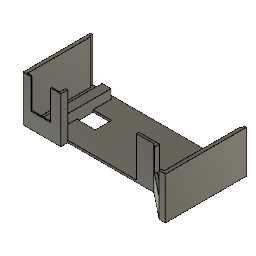
Box_gap_part1 v2 (Autodesk Fusion 360 design; units mm, degrees)
Autodesk Fusion 360 part; units mm, degrees
note: some values were not read from the file. Set by a fixed rule: which sketch regions a step uses.
sketch "草图1" plane through (0, 0, 0) normal (0, 1, 0) x (1, 0, 0)
  line L0 (0, 0) -> (56, 0)
  line L1 (56, 0) -> (56, -136)
  line L2 (56, -136) -> (0, -136)
  line L3 (0, -136) -> (0, 0)
  line L4 (3, -3) -> (53, -3)
  line L5 (53, -3) -> (53, -133)
  line L6 (53, -133) -> (3, -133)
  line L7 (3, -133) -> (3, -3)
  dimension "d1" = 136
  dimension "d2" = 56
  dimension "d3" = 3
  dimension "d4" = 3
  dimension "d5" = 3
  dimension "d6" = 3
  constraint horizontal L0
  constraint vertical L1
  constraint horizontal L2
  constraint vertical L3
  constraint coincident L0.start L3.end
  constraint horizontal L4
  constraint vertical L5
  constraint horizontal L6
  constraint vertical L7
  measures "d1" distance of L0.end L1.end
  measures "d2" distance of L1.end L2.end
  measures "d3" distance of L2 L6
  measures "d4" distance of L0 L4
  measures "d5" distance of L1 L5
  measures "d6" distance of L3 L7
extrude "拉伸1" add sketch "草图1" along normal blind 53
sketch "草图2" plane through (56, 0, 0) normal (1, 0, 0) x (0, 1, 0)
  line L0 (0, 136) -> (0, 0)
  line L1 (0, 0) -> (53, 0)
  line L2 (53, 0) -> (53, 136)
  line L3 (53, 136) -> (0, 136)
  line L4 (0, 0) -> (0, 28)
  line L5 (-16, 5) -> (0, 25)
  line L6 (0, 0) -> (-18, 0)
  line L7 (-18, 0) -> (-18, 5.5)
  line L8 (-18, 5.5) -> (0, 28)
  line L9 (0, 3) -> (-16, 3)
  line L10 (-16, 3) -> (-16, 5)
  point P0 (0, 3)
  dimension "d9" = 28
  dimension "d13" = 16
  dimension "d14" = 18
  constraint coincident L0.end L1.start
  constraint coincident L0 L4.end
  constraint perpendicular L1 L4
  constraint coincident L4 L5.end
  constraint perpendicular L4 L6
  constraint coincident P0 L9.start
  constraint perpendicular L4 L9
  measures "d9" distance of L0.end L4.end
  measures "d13" distance of P0 L9.end
  measures "d14" distance of L0.end L6.end
extrude "拉伸2" add sketch "草图2" against normal blind 56 contours L0 L4 L5 L6 L7 L8 L9 L10
sketch "草图3" plane through (0, 0, 0) normal (1, 0, 0) x (0, 1, 0)
  line L0 (0, 0) -> (0, 28)
  line L1 (0, 25) -> (0, 3)
  line L2 (-16, 3) -> (0, 3)
  line L3 (-16, 3) -> (-16, 5)
  line L4 (-16, 5) -> (0, 25)
  point P0 (0, 25)
  point P1 (0, 3)
  point P2 (-16, 3)
  point P3 (-16, 5)
  point P4 (0, 25)
  constraint coincident P4 P0
  constraint coincident P1 L1.end
  constraint coincident P2 L2.start
  constraint coincident P3 L3.end
extrude "拉伸3" add sketch "草图3" along normal blind 3
sketch "草图4" plane through (56, 0, 0) normal (1, 0, 0) x (0, 1, 0)
  line L0 (0, 25) -> (0, 3)
  line L1 (0, 3) -> (-16, 3)
  line L2 (-16, 3) -> (-16, 5)
  line L3 (-16, 5) -> (0, 25)
  line L4 (0, 28) -> (-18, 5.5)
  line L5 (-18, 5.5) -> (-18, 0)
  line L6 (-18, 0) -> (53, 0)
  line L7 (53, 0) -> (53, 136)
  line L8 (53, 136) -> (0, 136)
  line L9 (0, 136) -> (0, 28)
  line L10 (0, 25) -> (0, 3)
  line L11 (-16, 5) -> (0, 25)
  constraint coincident L0.start L3.end
  constraint coincident L0.end L1.start
  constraint coincident L2.end L3.start
extrude "拉伸4" add sketch "草图4" against normal blind 3 contours L0 L1 L2 L3 L10 L11
sketch "草图5" plane through (0, 0, 0) normal (0, -1, 0) x (1, 0, 0)
  line L0 (53, 28) -> (56, 28)
  line L1 (56, 28) -> (56, 136)
  line L2 (56, 136) -> (0, 136)
  line L3 (0, 136) -> (0, 28)
  line L4 (0, 28) -> (3, 28)
  line L5 (3, 28) -> (3, 133)
  line L6 (3, 133) -> (53, 133)
  line L7 (53, 133) -> (53, 28)
  line L8 (53, 25) -> (3, 25)
  line L9 (3, 25) -> (3, 45)
  line L10 (3, 45) -> (53, 45)
  line L11 (53, 45) -> (53, 25)
  point P0 (53, 25)
  dimension "d21" = 20
  constraint horizontal L8
  constraint vertical L9
  constraint horizontal L10
  constraint vertical L11
  constraint coincident L5 L9.end
  constraint coincident P0 L8.start
  measures "d21" distance of P0 L10.end
extrude "拉伸7" add sketch "草图5" against normal blind 2 contours L5 L7 L8 L9 L10 L11
extrude "拉伸5" add sketch "草图5" against normal blind 2 contours L5 L7 L8 L9 L10 L11
sketch "草图7" plane through (0, -18, 0) normal (0, -1, 0) x (1, 0, 0)
  line L0 (56, 0) -> (56, 5.5)
  line L1 (56, 5.5) -> (0, 5.5)
  line L2 (0, 5.5) -> (0, 0)
  line L3 (0, 0) -> (56, 0)
  line L4 (18, 3) -> (38, 3)
  line L5 (38, 3) -> (38, 25)
  line L6 (38, 25) -> (18, 25)
  line L7 (18, 25) -> (18, 3)
  line L8 (3, 3) -> (53, 3)
  line L9 (53, 25) -> (3, 25)
  dimension "d26" = 15
  dimension "d27" = 15
  constraint horizontal L4
  constraint vertical L5
  constraint horizontal L6
  constraint vertical L7
  constraint coincident L5.end L9
  constraint coincident L4.start L8
  measures "d26" distance of L4.start L8.start
  measures "d27" distance of L4.end L8.end
extrude "拉伸6" cut sketch "草图7" against normal blind 20 contours L1 L5 L6 L7 L9
sketch "草图8" plane through (56, 0, 0) normal (1, 0, 0) x (0, 1, 0)
  line L0 (0, 28) -> (-18, 5.5)
  line L1 (-18, 5.5) -> (-18, 0)
  line L2 (-18, 0) -> (53, 0)
  line L3 (53, 0) -> (53, 136)
  line L4 (53, 136) -> (0, 136)
  line L5 (0, 136) -> (0, 28)
  line L6 (0, 136) -> (-6, 136)
  line L7 (0, 133) -> (-5, 133)
  line L8 (-5, 133) -> (-5, 105)
  line L9 (-5, 105) -> (0, 105)
  line L10 (-6, 136) -> (-6, 103)
  line L11 (-6, 103) -> (0, 102.9799)
  point P0 (0, 136)
  point P1 (0, 133)
  dimension "d32" = 6
  dimension "d36" = 28
  dimension "d37" = 5
  dimension "d38" = 33
  constraint coincident P0 L4.end
  constraint perpendicular L5 L6
  constraint coincident P1 L7.start
  constraint perpendicular L5 L7
  constraint perpendicular L7 L8
  constraint coincident L5 L9.end
  constraint perpendicular L8 L9
  constraint perpendicular L6 L10
  constraint coincident L5 L11.end
  measures "d32" distance of L6.end P0
  measures "d36" distance of L7.end L8.end
  measures "d37" distance of L8 L9.end
  measures "d38" distance of L6.end L10.end
extrude "拉伸8" add sketch "草图8" against normal blind 56 contours L5 L6 L7 L8 L9 L10 L11
sketch "草图9" plane through (0, 0, 0) normal (-1, 0, 0) x (0, -1, 0)
  line L0 (0, 105) -> (0, 133)
  line L1 (0, 133) -> (5, 133)
  line L2 (5, 133) -> (5, 105)
  line L3 (5, 105) -> (0, 105)
  line L4 (0, 102.9799) -> (6, 103)
  line L5 (6, 103) -> (6, 136)
  line L6 (6, 136) -> (-53, 136)
  line L7 (-53, 136) -> (-53, 0)
  line L8 (-53, 0) -> (18, 0)
  line L9 (18, 0) -> (18, 5.5)
  line L10 (18, 5.5) -> (0, 28)
  line L11 (0, 28) -> (0, 102.9799)
  line L12 (0, 133) -> (5, 133)
  line L13 (5, 133) -> (5, 105)
  line L14 (5, 105) -> (0, 105)
  line L15 (0, 105) -> (0, 133)
  constraint horizontal L12
  constraint vertical L13
  constraint horizontal L14
  constraint vertical L15
  constraint coincident L2.end L3.start
  constraint coincident L0.end L1.start
extrude "拉伸9" add sketch "草图9" against normal blind 3 contours L0 L1 L2 L3 L12 L13 L14 L15
sketch "草图10" plane through (56, 0, 0) normal (1, 0, 0) x (0, 1, 0)
  line L0 (0, 102.9799) -> (0, 28)
  line L1 (0, 28) -> (-18, 5.5)
  line L2 (-18, 5.5) -> (-18, 0)
  line L3 (-18, 0) -> (53, 0)
  line L4 (53, 0) -> (53, 136)
  line L5 (53, 136) -> (-6, 136)
  line L6 (-6, 136) -> (-6, 103)
  line L7 (-6, 103) -> (0, 102.9799)
  line L8 (0, 105) -> (-5, 105)
  line L9 (-5, 105) -> (-5, 133)
  line L10 (-5, 133) -> (0, 133)
  line L11 (0, 133) -> (0, 105)
  line L12 (0, 133) -> (-5, 133)
  line L13 (-5, 133) -> (-5, 105)
  line L14 (-5, 105) -> (0, 105)
  line L15 (0, 105) -> (0, 133)
  constraint horizontal L12
  constraint vertical L13
  constraint horizontal L14
  constraint vertical L15
  constraint coincident L8.end L9.start
  constraint coincident L10.end L11.start
extrude "拉伸10" add sketch "草图10" against normal blind 3 contours L8 L9 L10 L11 L12 L13 L14 L15
sketch "草图11" plane through (0, -6, 0) normal (0, -1, 0) x (1, 0, 0)
  line L0 (56, 103) -> (56, 136)
  line L1 (56, 136) -> (0, 136)
  line L2 (0, 136) -> (0, 103)
  line L3 (0, 103) -> (56, 103)
  line L4 (41, 129) -> (15, 129)
  line L5 (15, 129) -> (15, 112)
  line L6 (15, 112) -> (41, 112)
  line L7 (41, 112) -> (41, 129)
  dimension "d45" = 7
  dimension "d46" = 15
  dimension "d47" = 15
  dimension "d48" = 17
  constraint horizontal L4
  constraint vertical L5
  constraint horizontal L6
  constraint vertical L7
  measures "d45" distance of L1 L4
  measures "d46" distance of L0 L7
  measures "d47" distance of L2 L5
  measures "d48" distance of L4.start L6.end
extrude "拉伸11" cut sketch "草图11" against normal blind 1 contours L4 L5 L6 L7
sketch "草图12" plane through (0, 0, 0) normal (0, -1, 0) x (1, 0, 0)
  line L0 (56, 102.9799) -> (53, 102.9799)
  line L1 (53, 102.9799) -> (53, 45)
  line L2 (53, 45) -> (3, 45)
  line L3 (3, 45) -> (3, 102.9799)
  line L4 (3, 102.9799) -> (0, 102.9799)
  line L5 (0, 102.9799) -> (0, 28)
  line L6 (0, 28) -> (56, 28)
  line L7 (56, 28) -> (56, 102.9799)
  line L8 (53, 45) -> (3, 45)
  line L9 (3, 45) -> (3, 43)
  line L10 (3, 43) -> (53, 43)
  line L11 (53, 43) -> (53, 45)
  line L12 (3, 45) -> (3, 25)
  dimension "d51" = 2
  constraint horizontal L8
  constraint vertical L9
  constraint horizontal L10
  constraint vertical L11
  constraint coincident L9.end L12
  constraint coincident L1.end L2.start
  measures "d51" distance of L1.end L10.end
extrude "拉伸12" cut sketch "草图12" against normal blind 3 contours L2 L8 L9 L10 L11 L12
sketch "草图13" plane through (56, 0, 0) normal (1, 0, 0) x (0, 1, 0)
  line L0 (0, 102.9799) -> (0, 28)
  line L1 (0, 28) -> (-18, 5.5)
  line L2 (-18, 5.5) -> (-18, 0)
  line L3 (-18, 0) -> (53, 0)
  line L4 (53, 0) -> (53, 136)
  line L5 (53, 136) -> (-6, 136)
  line L6 (-6, 136) -> (-6, 103)
  line L7 (-6, 103) -> (0, 102.9799)
  line L8 (0, 102.9799) -> (14, 102.9799)
  line L9 (14, 102.9799) -> (14, 88.9799)
  line L10 (14, 88.9799) -> (0, 88.9799)
  line L11 (0, 88.9799) -> (0, 102.9799)
  line L12 (14, 102.9799) -> (17, 102.9799)
  line L13 (17, 102.9799) -> (14, 102.9799)
  line L14 (14, 102.9799) -> (14, 88.9799)
  line L15 (14, 88.9799) -> (17, 88.9799)
  line L16 (17, 88.9799) -> (17, 102.9799)
  dimension "d54" = 14
  dimension "d55" = 14
  dimension "d56" = 3
  constraint horizontal L8
  constraint vertical L9
  constraint horizontal L10
  constraint vertical L11
  constraint coincident L0.start L7.end
  constraint perpendicular L9 L12
  constraint horizontal L13
  constraint vertical L14
  constraint horizontal L15
  constraint vertical L16
  measures "d54" distance of L0.start L8.end
  measures "d55" distance of L0.start L10.end
  measures "d56" distance of L8.end L12.end
extrude "拉伸13" cut sketch "草图13" against normal blind 3 contours L9 L12 L13 L14 L15 L16
sketch "草图14" plane through (56, 0, 0) normal (1, 0, 0) x (0, 1, 0)
  line L0 (14, 102.9799) -> (17, 102.9799)
  line L1 (17, 102.9799) -> (17, 88.9799)
  line L2 (17, 88.9799) -> (14, 88.9799)
  line L3 (14, 88.9799) -> (14, 102.9799)
  line L4 (0, 102.9799) -> (0, 28)
  line L5 (0, 28) -> (-18, 5.5)
  line L6 (-18, 5.5) -> (-18, 0)
  line L7 (-18, 0) -> (53, 0)
  line L8 (53, 0) -> (53, 136)
  line L9 (53, 136) -> (-6, 136)
  line L10 (-6, 136) -> (-6, 103)
  line L11 (-6, 103) -> (0, 102.9799)
  line L12 (53, 136) -> (-18, 136)
  line L13 (-18, 136) -> (-18, 0)
  line L14 (-18, 0) -> (53, 0)
  line L15 (53, 0) -> (53, 136)
  constraint horizontal L12
  constraint vertical L13
  constraint horizontal L14
  constraint vertical L15
  constraint coincident L6.end L7.start
  constraint coincident L8.end L9.start
extrude "拉伸14" cut sketch "草图14" against normal blind 1 contours L4 L5 L6 L7 L8 L9 L10 L11 L12 L13 L14 L15
sketch "草图15" plane through (0, 0, 0) normal (-1, 0, 0) x (0, -1, 0)
  line L0 (0, 102.9799) -> (6, 103)
  line L1 (6, 103) -> (6, 136)
  line L2 (6, 136) -> (-53, 136)
  line L3 (-53, 136) -> (-53, 0)
  line L4 (-53, 0) -> (18, 0)
  line L5 (18, 0) -> (18, 5.5)
  line L6 (18, 5.5) -> (0, 28)
  line L7 (0, 28) -> (0, 102.9799)
  line L8 (-53, 136) -> (18, 136)
  line L9 (18, 136) -> (18, 0)
  line L10 (18, 0) -> (-53, 0)
  line L11 (-53, 0) -> (-53, 136)
  constraint horizontal L8
  constraint vertical L9
  constraint horizontal L10
  constraint vertical L11
  constraint coincident L4.end L5.start
  constraint coincident L2.end L3.start
extrude "拉伸15" cut sketch "草图15" against normal blind 1 contours L0 L1 L2 L3 L4 L5 L6 L7 L8 L9 L10 L11
sketch "草图16" plane through (55, 0, 0) normal (1, 0, 0) x (0, 1, 0)
  line L0 (17, 88.9799) -> (14, 88.9799)
  line L1 (14, 88.9799) -> (14, 102.9799)
  line L2 (14, 102.9799) -> (17, 102.9799)
  line L3 (17, 102.9799) -> (17, 88.9799)
  line L4 (53, 0) -> (53, 136)
  line L5 (53, 136) -> (-6, 136)
  line L6 (-6, 136) -> (-6, 103)
  line L7 (-6, 103) -> (0, 102.9799)
  line L8 (0, 102.9799) -> (0, 28)
  line L9 (0, 28) -> (-18, 5.5)
  line L10 (-18, 5.5) -> (-18, 0)
  line L11 (-18, 0) -> (53, 0)
  line L12 (0, 102.9799) -> (14, 102.9799)
  line L13 (14, 102.9799) -> (14, 54.9799)
  line L14 (14, 54.9799) -> (0, 54.9799)
  line L15 (0, 54.9799) -> (0, 102.9799)
  line L16 (14, 54.9799) -> (22, 54.9799)
  line L17 (22, 54.9799) -> (22, 40.9799)
  line L18 (22, 40.9799) -> (14, 40.9799)
  line L19 (14, 40.9799) -> (14, 54.9799)
  dimension "d63" = 48
  dimension "d64" = 14
  dimension "d65" = 14
  dimension "d66" = 8
  constraint horizontal L12
  constraint vertical L13
  constraint horizontal L14
  constraint vertical L15
  constraint coincident L7.end L8.start
  constraint horizontal L16
  constraint vertical L17
  constraint horizontal L18
  constraint vertical L19
  measures "d63" distance of L1.end L13.end
  measures "d64" distance of L7.end L1.end
  measures "d65" distance of L16.end L17.end
  measures "d66" distance of L13.end L16.end
extrude "拉伸16" cut sketch "草图16" against normal blind 2 contours L16 L17 L18 L19
sketch "草图17" plane through (1, 0, 0) normal (-1, 0, 0) x (0, -1, 0)
  line L0 (18, 5.5) -> (0, 28)
  line L1 (0, 28) -> (0, 102.9799)
  line L2 (0, 102.9799) -> (6, 103)
  line L3 (6, 103) -> (6, 136)
  line L4 (6, 136) -> (-53, 136)
  line L5 (-53, 136) -> (-53, 0)
  line L6 (-53, 0) -> (18, 0)
  line L7 (18, 0) -> (18, 5.5)
  line L8 (6, 136) -> (-20, 136)
  line L9 (-20, 136) -> (-20, 115)
  line L10 (-20, 115) -> (6, 115)
  line L11 (6, 115) -> (6, 136)
  line L12 (-20, 115) -> (-34, 115)
  line L13 (-34, 115) -> (-34, 99)
  line L14 (-34, 99) -> (-20, 99)
  line L15 (-20, 99) -> (-20, 115)
  dimension "d69" = 26
  dimension "d70" = 21
  dimension "d71" = 14
  dimension "d72" = 16
  constraint horizontal L8
  constraint vertical L9
  constraint horizontal L10
  constraint vertical L11
  constraint coincident L3.end L4.start
  constraint horizontal L12
  constraint vertical L13
  constraint horizontal L14
  constraint vertical L15
  measures "d69" distance of L3.end L8.end
  measures "d70" distance of L3.end L10.end
  measures "d71" distance of L9.end L12.end
  measures "d72" distance of L9.end L14.end
extrude "拉伸17" cut sketch "草图17" against normal blind 2 contours L12 L13 L14 L15
sketch "草图18" plane through (55, 0, 0) normal (1, 0, 0) x (0, 1, 0)
  line L0 (22, 54.9799) -> (22, 40.9799)
  line L1 (22, 40.9799) -> (14, 40.9799)
  line L2 (14, 40.9799) -> (14, 54.9799)
  line L3 (14, 54.9799) -> (22, 54.9799)
  line L4 (17, 88.9799) -> (14, 88.9799)
  line L5 (14, 88.9799) -> (14, 102.9799)
  line L6 (14, 102.9799) -> (17, 102.9799)
  line L7 (17, 102.9799) -> (17, 88.9799)
  line L8 (53, 0) -> (53, 136)
  line L9 (53, 136) -> (-6, 136)
  line L10 (-6, 136) -> (-6, 103)
  line L11 (-6, 103) -> (0, 102.9799)
  line L12 (0, 102.9799) -> (0, 28)
  line L13 (0, 28) -> (-18, 5.5)
  line L14 (-18, 5.5) -> (-18, 0)
  line L15 (-18, 0) -> (53, 0)
  line L16 (53, 136) -> (-18, 136)
  line L17 (-18, 136) -> (-18, 0)
  line L18 (-18, 0) -> (53, 0)
  line L19 (53, 0) -> (53, 136)
  constraint horizontal L16
  constraint vertical L17
  constraint horizontal L18
  constraint vertical L19
  constraint coincident L14.end L15.start
  constraint coincident L8.end L9.start
sketch "草图19" plane through (1, 0, 0) normal (-1, 0, 0) x (0, -1, 0)
  line L0 (-34, 115) -> (-20, 115)
  line L1 (-20, 115) -> (-20, 99)
  line L2 (-20, 99) -> (-34, 99)
  line L3 (-34, 99) -> (-34, 115)
  line L4 (18, 5.5) -> (0, 28)
  line L5 (0, 28) -> (0, 102.9799)
  line L6 (0, 102.9799) -> (6, 103)
  line L7 (6, 103) -> (6, 136)
  line L8 (6, 136) -> (-53, 136)
  line L9 (-53, 136) -> (-53, 0)
  line L10 (-53, 0) -> (18, 0)
  line L11 (18, 0) -> (18, 5.5)
  line L12 (-53, 136) -> (18, 136)
  line L13 (18, 136) -> (18, 0)
  line L14 (18, 0) -> (-53, 0)
  line L15 (-53, 0) -> (-53, 136)
  constraint horizontal L12
  constraint vertical L13
  constraint horizontal L14
  constraint vertical L15
  constraint coincident L10.end L11.start
  constraint coincident L8.end L9.start
sketch "草图20" plane through (0, 53, 0) normal (0, 1, 0) x (-1, 0, 0)
  line L0 (-1, 136) -> (-55, 136)
  line L1 (-55, 0) -> (-1, 0)
  line L2 (-53, 133) -> (-3, 133)
  line L3 (-3, 133) -> (-3, 3)
  line L4 (-3, 3) -> (-53, 3)
  line L5 (-53, 3) -> (-53, 133)
  line L6 (-3, 105) -> (-11, 105)
  line L7 (-11, 105) -> (-11, 115)
  line L8 (-11, 115) -> (-3, 115)
  line L9 (-3, 115) -> (-3, 105)
  line L10 (-11, 115) -> (-3, 115)
  line L11 (-3, 115) -> (-3, 123)
  line L12 (-3, 123) -> (-11, 123)
  line L13 (-11, 123) -> (-11, 115)
  line L14 (-55, 136) -> (-55, 0)
  line L15 (-1, 0) -> (-1, 136)
  point P0 (-3, 105)
  dimension "d79" = 8
  dimension "d80" = 10
  dimension "d81" = 8
  constraint horizontal L6
  constraint vertical L7
  constraint horizontal L8
  constraint vertical L9
  constraint coincident P0 L6.start
  constraint horizontal L10
  constraint vertical L11
  constraint horizontal L12
  constraint vertical L13
  constraint coincident L3 L11.end
  measures "d79" distance of L7.end L8.end
  measures "d80" distance of L6.end L7.end
  measures "d81" distance of L7.end L12.end
extrude "拉伸20" add sketch "草图20" against normal blind 58 contours L3 L8 L10 L11 L12 L13
sketch "草图21" plane through (0, 53, 0) normal (0, 1, 0) x (-1, 0, 0)
  line L0 (-1, 136) -> (-55, 136)
  line L1 (-55, 0) -> (-1, 0)
  line L2 (-53, 133) -> (-3, 133)
  line L3 (-3, 133) -> (-3, 123)
  line L4 (-3, 123) -> (-11, 123)
  line L5 (-11, 123) -> (-11, 115)
  line L6 (-11, 115) -> (-3, 115)
  line L7 (-3, 115) -> (-3, 3)
  line L8 (-3, 3) -> (-53, 3)
  line L9 (-53, 3) -> (-53, 133)
  line L10 (-53, 104.9587) -> (-45, 104.9587)
  line L11 (-45, 104.9587) -> (-45, 114.9587)
  line L12 (-45, 114.9587) -> (-53, 114.9587)
  line L13 (-53, 114.9587) -> (-53, 104.9587)
  line L14 (-45, 114.9587) -> (-53, 114.9587)
  line L15 (-53, 114.9587) -> (-53, 122.9587)
  line L16 (-53, 122.9587) -> (-45, 122.9587)
  line L17 (-45, 122.9587) -> (-45, 114.9587)
  line L18 (-55, 136) -> (-55, 0)
  line L19 (-1, 0) -> (-1, 136)
  dimension "d85" = 10
  dimension "d86" = 8
  dimension "d87" = 8
  constraint horizontal L10
  constraint vertical L11
  constraint horizontal L12
  constraint vertical L13
  constraint coincident L9 L10.start
  constraint horizontal L14
  constraint vertical L15
  constraint horizontal L16
  constraint vertical L17
  constraint coincident L9 L15.end
  measures "d85" distance of L10.end L11.end
  measures "d86" distance of L15.end L16.end
  measures "d87" distance of L11.end L16.end
extrude "拉伸21" add sketch "草图21" against normal blind 58 contours L9 L12 L14 L15 L16 L17
sketch "草图22" plane through (0, 53, 0) normal (0, 1, 0) x (-1, 0, 0)
  line L0 (-1, 136) -> (-55, 136)
  line L1 (-55, 0) -> (-1, 0)
  line L2 (-53, 133) -> (-3, 133)
  line L3 (-3, 133) -> (-3, 123)
  line L4 (-3, 123) -> (-11, 123)
  line L5 (-11, 123) -> (-11, 115)
  line L6 (-11, 115) -> (-3, 115)
  line L7 (-3, 3) -> (-53, 3)
  line L8 (-53, 3) -> (-53, 114.9587)
  line L9 (-53, 114.9587) -> (-45, 114.9587)
  line L10 (-45, 114.9587) -> (-45, 122.9587)
  line L11 (-45, 122.9587) -> (-53, 122.9587)
  line L12 (-55, 136) -> (-55, 0)
  line L13 (-3, 115) -> (-3, 3)
  line L14 (-53, 122.9587) -> (-53, 133)
  line L15 (-1, 0) -> (-1, 136)
  point P0 (-7, 119)
sketch "草图23" plane through (0, 53, 0) normal (0, 1, 0) x (-1, 0, 0)
  line L0 (-1, 136) -> (-55, 136)
  line L1 (-55, 0) -> (-1, 0)
  line L2 (-53, 133) -> (-3, 133)
  line L3 (-3, 133) -> (-3, 123)
  line L4 (-3, 123) -> (-11, 123)
  line L5 (-11, 123) -> (-11, 115)
  line L6 (-11, 115) -> (-3, 115)
  line L7 (-3, 3) -> (-53, 3)
  line L8 (-53, 3) -> (-53, 114.9587)
  line L9 (-53, 114.9587) -> (-45, 114.9587)
  line L10 (-45, 114.9587) -> (-45, 122.9587)
  line L11 (-45, 122.9587) -> (-53, 122.9587)
  line L12 (-55, 136) -> (-55, 0)
  line L13 (-3, 115) -> (-3, 3)
  line L14 (-53, 122.9587) -> (-53, 133)
  line L15 (-1, 0) -> (-1, 136)
  point P0 (-49, 118.9587)
  dimension "d93" = 4
  dimension "d94" = 4
  measures "d93" distance of L10 P0
  measures "d94" distance of L11 P0
sketch "草图24" plane through (0, 53, 0) normal (0, 1, 0) x (-1, 0, 0)
  line L0 (-1, 136) -> (-55, 136)
  line L1 (-55, 0) -> (-1, 0)
  line L2 (-53, 133) -> (-3, 133)
  line L3 (-3, 133) -> (-3, 123)
  line L4 (-3, 123) -> (-11, 123)
  line L5 (-11, 123) -> (-11, 115)
  line L6 (-11, 115) -> (-3, 115)
  line L7 (-3, 3) -> (-53, 3)
  line L8 (-53, 3) -> (-53, 114.9587)
  line L9 (-53, 114.9587) -> (-45, 114.9587)
  line L10 (-45, 114.9587) -> (-45, 122.9587)
  line L11 (-45, 122.9587) -> (-53, 122.9587)
  line L12 (-3, 3) -> (-11, 3)
  line L13 (-11, 3) -> (-11, 11)
  line L14 (-11, 11) -> (-3, 11)
  line L15 (-3, 11) -> (-3, 3)
  line L16 (-55, 136) -> (-55, 0)
  line L17 (-3, 115) -> (-3, 3)
  line L18 (-53, 122.9587) -> (-53, 133)
  line L19 (-1, 0) -> (-1, 136)
  dimension "d98" = 8
  dimension "d99" = 8
  constraint horizontal L12
  constraint vertical L13
  constraint horizontal L14
  constraint vertical L15
  constraint coincident L7.start L12.start
  measures "d98" distance of L13.end L14.end
  measures "d99" distance of L12.end L13.end
extrude "拉伸22" add sketch "草图24" against normal blind 58 contours L7 L12 L13 L14 L15 L17
sketch "草图25" plane through (0, 53, 0) normal (0, 1, 0) x (-1, 0, 0)
  line L0 (-1, 136) -> (-55, 136)
  line L1 (-55, 0) -> (-1, 0)
  line L2 (-53, 133) -> (-3, 133)
  line L3 (-3, 133) -> (-3, 123)
  line L4 (-3, 123) -> (-11, 123)
  line L5 (-11, 123) -> (-11, 115)
  line L6 (-11, 115) -> (-3, 115)
  line L7 (-3, 11) -> (-11, 11)
  line L8 (-11, 11) -> (-11, 3)
  line L9 (-11, 3) -> (-53, 3)
  line L10 (-53, 3) -> (-53, 114.9587)
  line L11 (-53, 114.9587) -> (-45, 114.9587)
  line L12 (-45, 114.9587) -> (-45, 122.9587)
  line L13 (-45, 122.9587) -> (-53, 122.9587)
  line L14 (-53, 3) -> (-45, 3)
  line L15 (-45, 3) -> (-45, 11)
  line L16 (-45, 11) -> (-53, 11)
  line L17 (-53, 11) -> (-53, 3)
  line L18 (-55, 136) -> (-55, 0)
  line L19 (-1, 0) -> (-1, 136)
  line L20 (-3, 115) -> (-3, 11)
  line L21 (-53, 122.9587) -> (-53, 133)
  dimension "d102" = 8
  dimension "d103" = 8
  constraint horizontal L14
  constraint vertical L15
  constraint horizontal L16
  constraint vertical L17
  constraint coincident L9.end L10.start
  measures "d102" distance of L14.end L15.end
  measures "d103" distance of L15.end L16.end
extrude "拉伸23" add sketch "草图25" against normal blind 58 contours L9 L10 L14 L15 L16 L17
sketch "草图26" plane through (0, 53, 0) normal (0, 1, 0) x (-1, 0, 0)
  line L0 (-1, 136) -> (-55, 136)
  line L1 (-55, 0) -> (-1, 0)
  line L2 (-53, 133) -> (-3, 133)
  line L3 (-3, 133) -> (-3, 123)
  line L4 (-3, 123) -> (-11, 123)
  line L5 (-11, 123) -> (-11, 115)
  line L6 (-11, 115) -> (-3, 115)
  line L7 (-3, 115) -> (-3, 11)
  line L8 (-3, 11) -> (-11, 11)
  line L9 (-11, 11) -> (-11, 3)
  line L10 (-11, 3) -> (-45, 3)
  line L11 (-45, 3) -> (-45, 11)
  line L12 (-45, 11) -> (-53, 11)
  line L13 (-53, 11) -> (-53, 114.9587)
  line L14 (-53, 114.9587) -> (-45, 114.9587)
  line L15 (-45, 114.9587) -> (-45, 122.9587)
  line L16 (-45, 122.9587) -> (-53, 122.9587)
  line L17 (-53, 122.9587) -> (-53, 133)
  line L18 (-55, 136) -> (-55, 0)
  line L19 (-1, 0) -> (-1, 136)
  point P0 (-7, 7)
sketch "草图27" plane through (0, 53, 0) normal (0, 1, 0) x (-1, 0, 0)
  line L0 (-1, 136) -> (-55, 136)
  line L1 (-55, 0) -> (-1, 0)
  line L2 (-53, 133) -> (-3, 133)
  line L3 (-3, 133) -> (-3, 123)
  line L4 (-3, 123) -> (-11, 123)
  line L5 (-11, 123) -> (-11, 115)
  line L6 (-11, 115) -> (-3, 115)
  line L7 (-3, 115) -> (-3, 11)
  line L8 (-3, 11) -> (-11, 11)
  line L9 (-11, 11) -> (-11, 3)
  line L10 (-11, 3) -> (-45, 3)
  line L11 (-45, 3) -> (-45, 11)
  line L12 (-45, 11) -> (-53, 11)
  line L13 (-53, 11) -> (-53, 114.9587)
  line L14 (-53, 114.9587) -> (-45, 114.9587)
  line L15 (-45, 114.9587) -> (-45, 122.9587)
  line L16 (-45, 122.9587) -> (-53, 122.9587)
  line L17 (-53, 122.9587) -> (-53, 133)
  line L18 (-55, 136) -> (-55, 0)
  line L19 (-1, 0) -> (-1, 136)
  point P0 (-49, 7)
  dimension "d109" = 4
  dimension "d110" = 4
  measures "d109" distance of L11 P0
  measures "d110" distance of L12 P0
sketch "草图28" plane through (0, 53, 0) normal (0, 1, 0) x (-1, 0, 0)
  line L0 (-1, 0) -> (-1, 136)
  line L1 (-1, 136) -> (-55, 136)
  line L2 (-55, 136) -> (-55, 0)
  line L3 (-55, 0) -> (-1, 0)
  line L4 (-53, 133) -> (-3, 133)
  line L5 (-3, 133) -> (-3, 123)
  line L6 (-3, 123) -> (-11, 123)
  line L7 (-11, 123) -> (-11, 115)
  line L8 (-11, 115) -> (-3, 115)
  line L9 (-3, 115) -> (-3, 11)
  line L10 (-3, 11) -> (-11, 11)
  line L11 (-11, 11) -> (-11, 3)
  line L12 (-11, 3) -> (-45, 3)
  line L13 (-45, 3) -> (-45, 11)
  line L14 (-45, 11) -> (-53, 11)
  line L15 (-53, 11) -> (-53, 114.9587)
  line L16 (-53, 114.9587) -> (-45, 114.9587)
  line L17 (-45, 114.9587) -> (-45, 122.9587)
  line L18 (-45, 122.9587) -> (-53, 122.9587)
  line L19 (-53, 122.9587) -> (-53, 133)
  line L20 (-53, 134) -> (-3, 134)
  line L21 (-3, 134) -> (-3, 2)
  line L22 (-3, 2) -> (-53, 2)
  line L23 (-53, 2) -> (-53, 134)
  dimension "d114" = 2
  dimension "d115" = 50
  dimension "d116" = 2
  constraint horizontal L20
  constraint vertical L21
  constraint horizontal L22
  constraint vertical L23
  measures "d114" distance of L3 L22
  measures "d115" distance of L20.start L20.end
  measures "d116" distance of L1 L20
extrude "拉伸24" cut sketch "草图28" against normal blind 3 contours L4 L20 L21 L23 | L16 L17 L18 L23 | L6 L7 L8 L21 | L10 L11 L12 L13 L14 L21 L22 L23
sketch "草图29" plane through (55, 0, 0) normal (1, 0, 0) x (0, 1, 0)
  line L0 (22, 54.9799) -> (22, 40.9799)
  line L1 (22, 40.9799) -> (14, 40.9799)
  line L2 (14, 40.9799) -> (14, 54.9799)
  line L3 (14, 54.9799) -> (22, 54.9799)
  line L4 (17, 88.9799) -> (14, 88.9799)
  line L5 (14, 88.9799) -> (14, 102.9799)
  line L6 (14, 102.9799) -> (17, 102.9799)
  line L7 (17, 102.9799) -> (17, 88.9799)
  line L8 (53, 0) -> (53, 136)
  line L9 (53, 136) -> (-6, 136)
  line L10 (-6, 136) -> (-6, 103)
  line L11 (-6, 103) -> (0, 102.9799)
  line L12 (0, 102.9799) -> (0, 28)
  line L13 (0, 28) -> (-18, 5.5)
  line L14 (-18, 5.5) -> (-18, 0)
  line L15 (-18, 0) -> (53, 0)
  line L16 (-6, 136) -> (53, 136)
  line L17 (53, 136) -> (53, 73.0514)
  line L18 (53, 73.0514) -> (-6, 73.0514)
  line L19 (-6, 73.0514) -> (-6, 136)
  constraint horizontal L16
  constraint vertical L17
  constraint horizontal L18
  constraint vertical L19
  constraint coincident L8 L17.end
  constraint coincident L9.end L10.start
extrude "拉伸25" cut sketch "草图29" against normal blind 14 contours L8 L9 L10 L11 L12 L16 L17 L18 L19
sketch "草图30" plane through (55, 0, 0) normal (1, 0, 0) x (0, 1, 0)
  line L0 (53, 73.0514) -> (0, 73.0514)
  line L1 (0, 73.0514) -> (0, 28)
  line L2 (0, 28) -> (-18, 5.5)
  line L3 (-18, 5.5) -> (-18, 0)
  line L4 (-18, 0) -> (53, 0)
  line L5 (53, 0) -> (53, 73.0514)
  line L6 (22, 54.9799) -> (22, 40.9799)
  line L7 (22, 40.9799) -> (14, 40.9799)
  line L8 (14, 40.9799) -> (14, 54.9799)
  line L9 (14, 54.9799) -> (22, 54.9799)
  line L10 (-18, 0) -> (53, 0)
  line L11 (53, 0) -> (53, 73.0514)
  line L12 (53, 73.0514) -> (-18, 73.0514)
  line L13 (-18, 73.0514) -> (-18, 0)
  constraint horizontal L10
  constraint vertical L11
  constraint horizontal L12
  constraint vertical L13
  constraint coincident L0.start L5.end
  constraint coincident L3.end L4.start
extrude "拉伸26" cut sketch "草图30" against normal blind 17 contours L0 L1 L2 L3 L4 L5 L10 L11 L12 L13
move_body "移动1" bodies 1 to x (0, 0, 1) y (0, 1, 0) z (-1, 0, 0) at (66.5, -30, 4.5)
